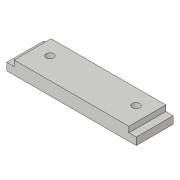
# Autodesk Inventor part: Lidar Sensor Case Piece 3
Saved by Autodesk Inventor 2018.3 (Build 223284000, 284)
## iProperties
Created: 2019-02-26
Part Number: Lidar Sensor Case Piece 3
Material: Generic
Document SubType Name: Modeling
Designer: aye06091
Mass: 4.62164 g
Surface Area: 26.1894 cm^2
Volume: 4.62164 cm^3
Density: 1 g/cm^3
Appearance: Default
Author: aye06091
Autodesk Inventor part; units mm, degrees
ref_plane "YZ Plane" through (0, 0, 0) normal (1, 0, 0) x (0, 1, 0)
ref_plane "XZ Plane" through (0, 0, 0) normal (0, 1, 0) x (-1, 0, 0)
ref_plane "XY Plane" through (0, 0, 0) normal (0, 0, 1) x (1, 0, 0)
sketch "Sketch1" plane through (0, 0, 0) normal (0, 1, 0) x (-1, 0, 0)
  line L0 (0, 0) -> (-55.6345, 0)
  line L1 (-55.6345, 0) -> (-55.6345, 15.875)
  line L2 (-55.6345, 15.875) -> (0, 15.875)
  line L3 (0, 15.875) -> (0, 0)
  dimension "d0" = 55.6345
  dimension "d1" = 15.875
  constraints: 8 end point, 2 parallel, 1 horizontal, 1 perpendicular
  measures "d0" distance of L0.start L0.end
  measures "d1" distance of L2.end L0.start
extrude "Extrusion1" add sketch "Sketch1" along normal blind 5.6134
sketch "Sketch7" plane through (0, 5.6134, 0) normal (0, 1, 0) x (1, 0, 0)
  circle A0 centre (9.3218, -6.6524) radius 1.6
  circle A1 centre (46.3218, -6.6524) radius 1.6
  line L0 (0, 0) -> (0, -15.875) projected
  line L1 (55.6345, 0) -> (0, 0) projected
  line L2 (55.6345, -15.875) -> (55.6345, 0) projected
  dimension "d22" = 3.2
  dimension "d23" = 3.2
  dimension "d24" = 37
  dimension "d43" = 6.6524
  dimension "d44" = 6.6524
  dimension "d48" = 9.3218
  dimension "d49" = 9.3127
  constraints: 2 centre point
  measures "d22" diameter of A0
  measures "d23" diameter of A1
  measures "d24" distance of A1.centre A0.centre
  measures "d43" distance from line of L1 A0.centre
  measures "d44" distance from line of L1 A1.centre
  measures "d48" distance from line of L0 A0.centre
  measures "d49" distance from line of L2 A1.centre
extrude "Extrusion6" cut sketch "Sketch7" against normal blind 25.4
sketch "Sketch8" plane through (0, 5.6134, 0) normal (0, 1, 0) x (1, 0, 0)
  line L0 (55.6345, 0) -> (0, 0) projected
  line L1 (0, 0) -> (0, -15.875) projected
  line L2 (55.6345, -15.875) -> (55.6345, 0) projected
  line L3 (0, -15.875) -> (3.175, -15.875)
  line L4 (3.175, -15.875) -> (3.175, 0)
  line L5 (3.175, 0) -> (0, 0)
  line L6 (0, 0) -> (0, -15.875)
  line L7 (55.6345, -15.875) -> (52.4595, -15.875)
  line L8 (52.4595, -15.875) -> (52.4595, 0)
  line L9 (52.4595, 0) -> (55.6345, 0)
  line L10 (55.6345, 0) -> (55.6345, -15.875)
  dimension "d34" = 3.175
  dimension "d35" = 3.175
  constraints: 16 end point, 4 parallel, 2 horizontal, 2 perpendicular, 2 point on line
  measures "d34" distance between parallel lines of L1 L4
  measures "d35" distance between parallel lines of L2 L8
extrude "Extrusion7" cut sketch "Sketch8" against normal blind 2.4384
equation "\"d23\" = d22"
body "Solid1"
